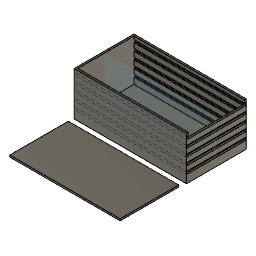
SP26_MindMasters_Enclosure_CameronVanOs (Autodesk Fusion 360 design; units mm, degrees)
part number: 2026-04-23-22-54-03-300
Autodesk Fusion 360 part; units mm, degrees
box "BoxPrimitive1" add length 96 width 180 height 70 placed x (0, 1, 0) y (-1, 0, 0) z (0, 0, 1) at (180, 0, 0) makes body 1
sketch "Sketch2" plane through (0, 0, 70) normal (0, 0, 1) x (-1, 0, 0)
  line L0 (-180, -96) -> (0, -96)
  line L1 (0, -96) -> (0, 0)
  line L2 (0, 0) -> (-180, 0)
  line L3 (-180, 0) -> (-180, -96)
  line L4 (-177, -3) -> (-177, -93)
  line L5 (-177, -93) -> (-3, -93)
  line L6 (-3, -93) -> (-3, -3)
  line L7 (-3, -3) -> (-177, -3)
  dimension "d6" = -3
extrude "Extrude1" cut sketch "Sketch2" against normal blind 67 contours L4 L5 L6 L7 bodies 1
sketch "Sketch3" plane through (180, 0, 0) normal (1, 0, 0) x (0, 1, 0)
  line L0 (0, 70) -> (0, 0)
  line L1 (0, 0) -> (96, 0)
  line L2 (96, 0) -> (96, 70)
  line L3 (96, 70) -> (0, 70)
  line L4 (3, 65) -> (1, 65)
  line L5 (1, 65) -> (1, 61)
  line L6 (1, 61) -> (3, 61)
  line L7 (3, 61) -> (3, 65)
  line L8 (93, 65) -> (95, 65)
  line L9 (95, 65) -> (95, 61)
  line L10 (95, 61) -> (93, 61)
  line L11 (93, 61) -> (93, 65)
  line L12 (3, 61) -> (93, 61)
  line L13 (93, 61) -> (93, 70)
  line L14 (93, 70) -> (3, 70)
  line L15 (3, 70) -> (3, 61)
  constraint horizontal L4
  constraint vertical L5
  constraint horizontal L6
  constraint vertical L7
  constraint horizontal L8
  constraint vertical L9
  constraint horizontal L10
  constraint vertical L11
  constraint horizontal L12
  constraint vertical L13
  constraint horizontal L14
  constraint vertical L15
  constraint coincident L3 L13.end
extrude "Extrude2" cut sketch "Sketch3" against normal blind 177 contours L3 L7 L11 L12 L13 L14 L15 | L4 L5 L6 L7 L15 | L8 L9 L10 L11 L13 bodies 1
move_body "Move1" bodies 1 to x (1, 0, 0) y (0, 1, 0) z (0, 0, 1) at (0, 150, 0)
sketch "Sketch4" plane through (0, 150, 0) normal (0, -1, 0) x (1, 0, 0)
  line L0 (0, 70) -> (0, 0)
  line L1 (0, 0) -> (180, 0)
  line L2 (180, 0) -> (180, 70)
  line L3 (180, 70) -> (0, 70)
box "BoxPrimitive2" add length 94 width 177 height 3 placed x (0, 1, 0) y (-1, 0, 0) z (0, 0, 1) at (177, 0, 0) separate body makes body 2
move_body "Move2" bodies 1 to x (1, 0, 0) y (0, 1, 0) z (0, 0, 1) at (-1.3962, -45.4644, 0)
sketch "Sketch6" plane through (178.6038, 0, 0) normal (1, 0, 0) x (0, 1, 0)
  line L0 (107.5356, 65) -> (107.5356, 70)
  line L1 (107.5356, 70) -> (104.5356, 70)
  line L2 (104.5356, 70) -> (104.5356, 0)
  line L3 (104.5356, 0) -> (200.5356, 0)
  line L4 (200.5356, 0) -> (200.5356, 70)
  line L5 (200.5356, 70) -> (197.5356, 70)
  line L6 (197.5356, 70) -> (197.5356, 65)
  line L7 (197.5356, 65) -> (199.5356, 65)
  line L8 (199.5356, 65) -> (199.5356, 61)
  line L9 (199.5356, 61) -> (105.5356, 61)
  line L10 (105.5356, 61) -> (105.5356, 65)
  line L11 (105.5356, 65) -> (107.5356, 65)
  line L12 (105.5356, 61) -> (104.5356, 61)
  line L13 (199.5356, 61) -> (200.5356, 61)
  line L14 (104.5356, 61) -> (200.5356, 61)
  line L15 (200.5356, 61) -> (200.5356, 0)
  line L16 (200.5356, 0) -> (104.5356, 0)
  line L17 (104.5356, 0) -> (104.5356, 61)
  line L18 (105.5356, 61) -> (105.5356, 0)
  line L19 (199.5356, 61) -> (199.5356, 0)
  line L20 (105.5356, 53) -> (199.5356, 53)
  line L21 (105.5356, 49) -> (199.5356, 49)
  line L22 (105.5356, 41) -> (199.5356, 41)
  line L23 (199.5356, 41) -> (199.5356, 37)
  line L24 (199.5356, 37) -> (105.5356, 37)
  line L25 (105.5356, 37) -> (105.5356, 41)
  line L26 (105.5356, 29) -> (199.5356, 29)
  line L27 (199.5356, 29) -> (199.5356, 25)
  line L28 (199.5356, 25) -> (105.5356, 25)
  line L29 (105.5356, 25) -> (105.5356, 29)
  line L30 (105.5356, 17) -> (200.5356, 17)
  line L31 (200.5356, 17) -> (200.5356, 13)
  line L32 (200.5356, 13) -> (105.5356, 13)
  line L33 (105.5356, 13) -> (105.5356, 17)
  dimension "d22" = 8
  dimension "d23" = 4
  dimension "d24" = 8
  dimension "d25" = 4
  dimension "d26" = 8
  dimension "d27" = 4
  dimension "d28" = 8
  dimension "d29" = 4
  dimension "d30" = 13
  constraint coincident L9.end L10.start
  constraint coincident L2 L12.end
  constraint perpendicular L2 L12
  constraint coincident L4 L13.end
  constraint perpendicular L4 L13
  constraint horizontal L14
  constraint vertical L15
  constraint horizontal L16
  constraint vertical L17
  constraint coincident L3.end L4.start
  constraint coincident L3 L18.end
  constraint perpendicular L3 L18
  constraint coincident L16 L19.end
  constraint perpendicular L16 L19
  constraint coincident L18 L20.start
  constraint coincident L19 L20.end
  constraint perpendicular L19 L20
  constraint coincident L18 L21.start
  constraint coincident L19 L21.end
  constraint perpendicular L19 L21
  constraint horizontal L22
  constraint vertical L23
  constraint horizontal L24
  constraint vertical L25
  constraint coincident L19 L23.end
  constraint coincident L18 L22.start
  constraint horizontal L26
  constraint vertical L27
  constraint horizontal L28
  constraint vertical L29
  constraint coincident L19 L27.end
  constraint coincident L18 L26.start
  constraint horizontal L30
  constraint vertical L31
  constraint horizontal L32
  constraint vertical L33
  constraint coincident L15 L31.end
  constraint coincident L18 L30.start
  measures "d22" distance of L14 L20
  measures "d23" distance of L20 L21
  measures "d24" distance of L21 L22
  measures "d25" distance of L22 L24
  measures "d26" distance of L24 L26
  measures "d27" distance of L26 L28
  measures "d28" distance of L28 L30
  measures "d29" distance of L30 L32
  measures "d30" distance of L16 L32
extrude "Extrude3" cut sketch "Sketch6" against normal blind 177 contours L18 L19 L20 L21 | L18 L19 L22 L23 L24 L25 | L18 L19 L30 L32 L33 | L18 L19 L26 L27 L28 L29 bodies 1
